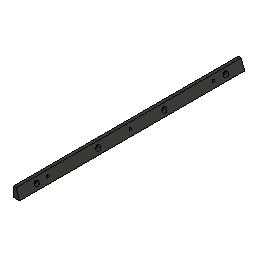
LED_wedge_left (Autodesk Fusion 360 design; units mm, degrees)
Autodesk Fusion 360 part; units mm, degrees
sketch "Skizze1" plane through (0, 0, 0) normal (0, 1, 0) x (1, 0, 0)
  line L0 (-29.0267, 0) -> (32.308, 0) construction
  line L1 (0, -25.3668) -> (0, 26.124) construction
  line L2 (0, 0) -> (0, -10)
  line L3 (0, -10) -> (-3, -10)
  line L4 (0, 0) -> (-6.815, 0)
  line L5 (-3, -10) -> (-6.815, 0)
  dimension "d1" = 10
  dimension "d2" = 6.815
  dimension "d3" = 3
  constraint horizontal L0
  constraint vertical L1
  constraint coincident L2.start L0
  constraint coincident L2.start L1
  constraint coincident L2.start L4.start
  constraint coincident L1 L2.end
  constraint perpendicular L2 L3
  constraint coincident L0 L4.end
  measures "d1" distance of L0 L2.end
  measures "d2" distance of L1 L4.end
  measures "d3" distance of L1 L3.end
extrude "Extrusion1" add sketch "Skizze1" along normal blind 238 makes body 1
sketch "Skizze2" plane through (0, 0, 0) normal (1, 0, 0) x (0, 1, 0)
  line L0 (0, 32.3505) -> (0, -25.958) construction
  line L1 (-11.6611, 0) -> (310, 0) construction
  line L2 (119, 63.4137) -> (119, -57.7153) construction
  line L3 (20, 43.9775) -> (20, -44.5265) construction
  line L4 (220, 51.6132) -> (220, -50) construction
  line L5 (85, 33.2182) -> (85, -47.6502) construction
  line L6 (155, 33.2182) -> (155, -42.444) construction
  line L7 (261.5293, 4.914) -> (-37.3941, 4.914) construction
  circle A0 centre (220, 4.914) radius 1.25
  circle A1 centre (220, 4.914) radius 2.5
  circle A2 centre (155, 4.914) radius 1.25
  circle A3 centre (155, 4.914) radius 2.5
  circle A4 centre (85, 4.914) radius 1.25
  circle A5 centre (85, 4.914) radius 2.5
  circle A6 centre (20, 4.914) radius 1.25
  circle A7 centre (20, 4.914) radius 2.5
  line L8 (207, 25.1754) -> (207, -27.1787) construction
  line L9 (32, 29.9975) -> (32, -45.4338) construction
  line L10 (257.1127, 6.878) -> (-52.1736, 6.878) construction
  line L11 (203.5, 0) -> (210.5, 0)
  line L12 (210.5, 0) -> (210.5, 6.878)
  line L13 (210.5, 6.878) -> (203.5, 6.878)
  line L14 (203.5, 6.878) -> (203.5, 0)
  line L15 (203.5, 0) -> (210.5, 6.878) construction
  line L16 (210.5, 0) -> (203.5, 6.878) construction
  line L17 (115.5, 0) -> (122.5, 0)
  line L18 (122.5, 0) -> (122.5, 6.878)
  line L19 (122.5, 6.878) -> (115.5, 6.878)
  line L20 (115.5, 6.878) -> (115.5, 0)
  line L21 (115.5, 0) -> (122.5, 6.878) construction
  line L22 (122.5, 0) -> (115.5, 6.878) construction
  line L23 (28.5, 0) -> (35.5, 0)
  line L24 (35.5, 0) -> (35.5, 6.878)
  line L25 (35.5, 6.878) -> (28.5, 6.878)
  line L26 (28.5, 6.878) -> (28.5, 0)
  line L27 (28.5, 0) -> (35.5, 6.878) construction
  line L28 (35.5, 0) -> (28.5, 6.878) construction
  point P0 (207, 3.439)
  point P1 (119, 3.439)
  point P2 (32, 3.439)
  dimension "d6" = 119
  dimension "d7" = 101
  dimension "d8" = 99
  dimension "d9" = 34
  dimension "d10" = 36
  dimension "d11" = 4.914
  dimension "d12" = 2.5
  dimension "d13" = 5
  dimension "d14" = 2.5
  dimension "d15" = 5
  dimension "d16" = 2.5
  dimension "d17" = 5
  dimension "d18" = 2.5
  dimension "d19" = 5
  dimension "d24" = 87
  dimension "d25" = 88
  dimension "d26" = 6.878
  dimension "d27" = 7
  dimension "d28" = 7
  dimension "d29" = 7
  constraint vertical L0
  constraint horizontal L1
  constraint coincident origin L0
  constraint coincident origin L1
  constraint perpendicular L1 L2
  constraint perpendicular L1 L3
  constraint perpendicular L1 L4
  constraint perpendicular L1 L5
  constraint perpendicular L1 L6
  constraint perpendicular L0 L7
  constraint coincident L4 A0.centre
  constraint coincident L7 A0.centre
  constraint concentric A0 A1
  constraint coincident L7 A2.centre
  constraint coincident L6 A2.centre
  constraint concentric A2 A3
  constraint coincident L5 A4.centre
  constraint coincident L7 A4.centre
  constraint concentric A4 A5
  constraint coincident L3 A6.centre
  constraint coincident L7 A6.centre
  constraint concentric A6 A7
  constraint perpendicular L7 L8
  constraint perpendicular L7 L9
  constraint perpendicular L3 L10
  constraint horizontal L11
  constraint perpendicular L11 L12
  constraint parallel L11 L13
  constraint parallel L12 L14
  constraint coincident L15 P0
  constraint coincident L16 P0
  constraint coincident L1 L11.start
  constraint coincident L8 P0
  constraint horizontal L17
  constraint perpendicular L17 L18
  constraint parallel L17 L19
  constraint parallel L18 L20
  constraint coincident L21 P1
  constraint coincident L22 P1
  constraint coincident L1 L17.start
  constraint coincident L2 P1
  constraint horizontal L23
  constraint perpendicular L23 L24
  constraint parallel L23 L25
  constraint parallel L24 L26
  constraint coincident L27 P2
  constraint coincident L28 P2
  constraint coincident L1 L23.start
  constraint coincident L9 P2
  constraint coincident L10 L13.end
  constraint coincident L10 L19.end
  constraint coincident L10 L24.end
  measures "d6" distance of L0 L2
  measures "d7" distance of L2 L4
  measures "d8" distance of L2 L3
  measures "d9" distance of L2 L5
  measures "d10" distance of L2 L6
  measures "d11" distance of L1 L7
  measures "d12" diameter of A6
  measures "d13" diameter of A7
  measures "d14" diameter of A4
  measures "d15" diameter of A5
  measures "d16" diameter of A2
  measures "d17" diameter of A3
  measures "d18" diameter of A0
  measures "d19" diameter of A1
  measures "d24" distance of L2 L9
  measures "d25" distance of L2 L8
  measures "d26" distance of L1 L10
  measures "d27" distance of L24 L26
  measures "d28" distance of L18 L20
  measures "d29" distance of L12 L14
extrude "Extrusion2" cut sketch "Skizze2" against normal blind 10 contours A0 | A1 | A2 | A3 | A4 | A5 | A6 | A7 bodies 1
extrude "Extrusion3" add sketch "Skizze2" against normal blind 2 contours A1 | A3 | A5 | A7 bodies 1
extrude "Extrusion4" add sketch "Skizze2" along normal blind 2 contours L11 L12 L13 L14 | L17 L18 L19 L20 | L23 L24 L25 L26 bodies 1
sketch "Skizze3" plane through (-5.9491, 0, 2.2696) normal (-0.934317, 0, 0.356442) x (0, -1, 0)
  ellipse E0 centre (-155, 2.8303) end of major axis (-155, 0.1546) minor radius 2.5
  ellipse E1 centre (-85, 2.8303) end of major axis (-85, 0.1546) minor radius 2.5
  ellipse E2 centre (-220, 2.8303) end of major axis (-220, 0.1546) minor radius 2.5
  ellipse E3 centre (-20, 2.8303) end of major axis (-20, 0.1546) minor radius 2.5
  line L0 (0, -2.4292) -> (0, 8.2738)
  line L1 (0, 8.2738) -> (-238, 8.2738)
  line L2 (-238, 8.2738) -> (-238, -2.4292)
  line L3 (-238, -2.4292) -> (0, -2.4292)
  line L4 (-256.1946, 8.2738) -> (13.3488, 8.2738) construction
  line L5 (-271.6873, 3.2738) -> (21.7349, 3.2738) construction
  line L6 (0, 76.206) -> (0, -63.9663) construction
  line L7 (-207, 69.0398) -> (-207, -61.5402) construction
  line L8 (-119, 70) -> (-119, -67.3252) construction
  line L9 (-32, 63.2186) -> (-32, -40) construction
  circle A0 centre (-207, 3.2738) radius 1.25
  circle A1 centre (-119, 3.2738) radius 1.25
  circle A2 centre (-32, 3.2738) radius 1.25
  line L10 (-205.7298, 1.0738) -> (-204.4597, 3.2738)
  line L11 (-204.4597, 3.2738) -> (-205.7298, 5.4738)
  line L12 (-205.7298, 5.4738) -> (-208.2702, 5.4738)
  line L13 (-208.2702, 5.4738) -> (-209.5403, 3.2738)
  line L14 (-209.5403, 3.2738) -> (-208.2702, 1.0738)
  line L15 (-208.2702, 1.0738) -> (-205.7298, 1.0738)
  line L16 (-117.7298, 1.0738) -> (-116.4597, 3.2738)
  line L17 (-116.4597, 3.2738) -> (-117.7298, 5.4738)
  line L18 (-117.7298, 5.4738) -> (-120.2702, 5.4738)
  line L19 (-120.2702, 5.4738) -> (-121.5403, 3.2738)
  line L20 (-121.5403, 3.2738) -> (-120.2702, 1.0738)
  line L21 (-120.2702, 1.0738) -> (-117.7298, 1.0738)
  line L22 (-30.7298, 1.0738) -> (-29.4597, 3.2738)
  line L23 (-29.4597, 3.2738) -> (-30.7298, 5.4738)
  line L24 (-30.7298, 5.4738) -> (-33.2702, 5.4738)
  line L25 (-33.2702, 5.4738) -> (-34.5403, 3.2738)
  line L26 (-34.5403, 3.2738) -> (-33.2702, 1.0738)
  line L27 (-33.2702, 1.0738) -> (-30.7298, 1.0738)
  point P0 (-207, 3.2738)
  point P1 (-119, 3.2738)
  point P2 (-32, 3.2738)
  dimension "d32" = 5
  dimension "d35" = 119
  dimension "d36" = 87
  dimension "d37" = 88
  dimension "d38" = 2.5
  dimension "d39" = 2.5
  dimension "d40" = 2.5
  dimension "d41" = 4.4
  dimension "d42" = 4.4
  dimension "d43" = 4.4
  constraint parallel L1 L4
  constraint coincident L1.end L4
  constraint perpendicular L2 L5
  constraint perpendicular L5 L6
  constraint coincident origin L6
  constraint vertical L7
  constraint perpendicular L3 L8
  constraint perpendicular L5 L9
  constraint coincident L5 P0
  constraint coincident L7 P0
  constraint coincident L5 P1
  constraint coincident L8 P1
  constraint coincident L5 P2
  constraint coincident P0 A0.centre
  constraint coincident P1 A1.centre
  constraint coincident P2 A2.centre
  constraint horizontal L15
  constraint horizontal L21
  constraint horizontal L27
  constraint coincident L9 P2
  measures "d32" distance of L4 L5
  measures "d35" distance of L6 L8
  measures "d36" distance of L8 L9
  measures "d37" distance of L7 L8
  measures "d38" diameter of A2
  measures "d39" diameter of A1
  measures "d40" diameter of A0
  measures "d41" distance of L24 L27
  measures "d42" distance of L18 L21
  measures "d43" distance of L12 L15
extrude "Extrusion5" cut sketch "Skizze3" against normal blind 8 contours A0 | A1 | A2 bodies 1
extrude "Extrusion6" cut sketch "Skizze3" against normal blind 3.8 contours L10 L11 L12 L13 L14 L15 | L16 L17 L18 L19 L20 L21 | L22 L23 L24 L25 L26 L27 bodies 1
extrude "Extrusion7" add sketch "Skizze3" against normal blind 2 contours L10 L11 L12 L13 L14 L15 | L16 L17 L18 L19 L20 L21 | L22 L23 L24 L25 L26 L27 bodies 1
mirror "Spiegeln1" about plane through (0, 0, 0) normal (1, 0, 0) of bodies 1 makes body 2
delete_body "Körper entfernen1" bodies 1
named bodies: "LED_wedge_left", "LED_wedge_right"
